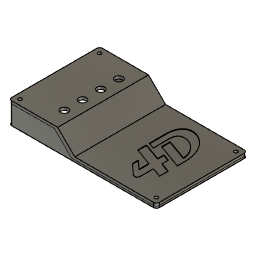
enclosure_top (Autodesk Fusion 360 design; units mm, degrees)
Autodesk Fusion 360 part; units mm, degrees
note: some values were not read from the file. Set by a fixed rule: which sketch regions a step uses.
sketch "Skizze1" plane through (0, 0, 0) normal (0, 0, 1) x (1, 0, 0)
  line L0 (0, 0) -> (130, 0)
  line L1 (130, 0) -> (130, 80)
  line L2 (130, 80) -> (0, 80)
  line L3 (0, 80) -> (0, 0)
  dimension "d1" = 80
  dimension "d2" = 130
  constraint horizontal L0
  constraint vertical L1
  constraint horizontal L2
  constraint vertical L3
  constraint coincident L0.start L3.end
  measures "d1" distance of L0.start L2.end
  measures "d2" distance of L0.start L0.end
extrude "Extrusion1" add sketch "Skizze1" along normal blind 19
sketch "Skizze2" plane through (0, 0, 0) normal (0, -1, 0) x (1, 0, 0)
  line L0 (0, 0) -> (130, 0)
  line L1 (130, 0) -> (130, 19)
  line L2 (130, 19) -> (0, 19)
  line L3 (0, 19) -> (0, 0)
  line L4 (0, 15) -> (40, 15)
  line L5 (40, 15) -> (55, 0)
  line L6 (55, 0) -> (0, 0)
  line L7 (0, 15) -> (0, 0)
  line L8 (43.0711, 19) -> (130, 19)
  line L9 (130, 19) -> (130, 4)
  line L10 (130, 4) -> (58.0711, 4)
  line L11 (58.0711, 4) -> (43.0711, 19)
  line L12 (47.5, 7.5) -> (51.0355, 11.0355) construction
  dimension "d5" = 15
  dimension "d6" = 40
  dimension "d7" = 45
  dimension "d8" = 135
  dimension "d10" = 4
  dimension "d11" = 5
  constraint coincident L3 L4.start
  constraint perpendicular L3 L4
  constraint coincident L0 L5.end
  constraint coincident L0.start L3.end
  constraint coincident L2 L8.start
  constraint coincident L1.end L2.start
  constraint perpendicular L1 L8
  constraint coincident L1 L9.end
  constraint perpendicular L8 L9
  constraint perpendicular L9 L10
  constraint midpoint L5 L12.start
  constraint perpendicular L5 L12
  constraint coincident L11 L12.end
  measures "d5" distance of L4.start L0.start
  measures "d6" distance of L4.start L4.end
  measures "d7" angle of L5 L6
  measures "d8" angle of L10 L11
  measures "d10" distance of L0.end L9.end
  measures "d11" distance of L12.start L12.end
extrude "Extrusion2" cut sketch "Skizze2" against normal blind 80 contours L0 L3 L4 L5 L6 L7 | L1 L2 L8 L9 L10 L11
shell "Schale1" thickness 2.5 removed faces 3 at (80, 53.3333, 0) at (45, 26.6667, 10) at (13.3333, 26.6667, 15)
sketch "Skizze3" plane through (0, 0, 0) normal (0, 0, -1) x (1, 0, 0)
  line L0 (127.5, -77.5) -> (55, -77.5)
  line L1 (55, -77.5) -> (55, -80)
  line L2 (55, -80) -> (130, -80)
  line L3 (130, -80) -> (130, 0)
  line L4 (130, 0) -> (55, 0)
  line L5 (55, 0) -> (55, -2.5)
  line L6 (55, -2.5) -> (127.5, -2.5)
  line L7 (127.5, -2.5) -> (127.5, -77.5)
  line L8 (55, 13.7) -> (135, 13.7)
  line L9 (135, 13.7) -> (135, -93.7)
  line L10 (135, -93.7) -> (55, -93.7)
  line L11 (55, -1.3) -> (127.5, -1.3)
  line L12 (128.7, -2.5) -> (128.7, -77.5)
  line L13 (127.5, -78.7) -> (55, -78.7)
  line L14 (55, 13.7) -> (55, -1.3)
  line L15 (55, -78.7) -> (55, -93.7)
  arc A0 (128.7, -2.5) -> (127.5, -1.3) centre (127.5, -2.5) ccw
  arc A1 (127.5, -78.7) -> (128.7, -77.5) centre (127.5, -77.5) ccw
  dimension "d16" = 1.3
  dimension "d17" = 1.3
  dimension "d20" = 1.3
  dimension "d21" = 15
  dimension "d22" = 80
  constraint horizontal L8
  constraint vertical L9
  constraint horizontal L10
  constraint horizontal L11
  constraint vertical L12
  constraint horizontal L13
  constraint vertical L14
  constraint vertical L15
  constraint vertical L11.start L13.end
  constraint equal L14 L15
  constraint coincident L5 L11.start
  constraint tangent L11 A0
  constraint tangent L12 A0
  constraint tangent L12 A1
  constraint tangent L13 A1
  constraint equal A0 A1
  constraint coincident L6.end L7.start
  measures "d16" distance of L4 L11.start
  measures "d17" distance of L1.end L13.end
  measures "d20" distance of L3 L12.start
  measures "d21" distance of L8.start L11.start
  measures "d22" distance of L8.start L8.end
extrude "Extrusion3" cut sketch "Skizze3" against normal blind 1.5 contours L1 L2 L3 L4 L5 L11 L12 L13 L14 L15 A0 A1
sketch "Skizze4" plane through (0, 0, 15) normal (0, 0, -1) x (1, 0, 0)
  line L0 (2.5, -77.5) -> (2.5, -2.5)
  line L1 (0, 0) -> (0, -80)
  line L2 (40, 8.7) -> (-10, 8.7)
  line L3 (-10, 8.7) -> (-10, -88.7)
  line L4 (-10, -88.7) -> (40, -88.7)
  line L5 (2.5, -1.3) -> (40, -1.3)
  line L6 (40, -78.7) -> (2.5, -78.7)
  line L7 (1.3, -77.5) -> (1.3, -2.5)
  line L8 (40, 8.7) -> (40, -1.3)
  line L9 (40, -88.7) -> (40, -78.7)
  line L10 (40, 0) -> (55, 0)
  line L11 (55, -80) -> (40, -80)
  arc A0 (2.5, -1.3) -> (1.3, -2.5) centre (2.5, -2.5) ccw
  arc A1 (1.3, -77.5) -> (2.5, -78.7) centre (2.5, -77.5) ccw
  point P0 (40, -2.5)
  dimension "d75" = 1.3
  dimension "d76" = 1.3
  dimension "d77" = 1.3
  dimension "d79" = 50
  dimension "d80" = 10
  constraint horizontal L2
  constraint vertical L3
  constraint horizontal L4
  constraint horizontal L5
  constraint horizontal L6
  constraint vertical L7
  constraint vertical L8
  constraint vertical L9
  constraint vertical L5.end L6.start
  constraint coincident L8 P0
  constraint tangent L5 A0
  constraint tangent L7 A0
  constraint tangent L6 A1
  constraint tangent L7 A1
  constraint equal A0 A1
  constraint coincident L0.end A0.centre
  constraint equal L8 L9
  measures "d75" distance of L5.end L10
  measures "d76" distance of L6.start L11
  measures "d77" distance of L1.start L7
  measures "d79" distance of L2.start L2.end
  measures "d80" distance of L2.start L5.end
extrude "Extrusion4" cut sketch "Skizze4" against normal blind 1.5
sketch "Skizze6" plane through (0, 80, 0) normal (0, 1, 0) x (-1, 0, 0)
  line L0 (-130, 1.5) -> (-55, 1.5)
  line L1 (-55, 1.5) -> (-55, 0)
  line L2 (-55, 0) -> (-40, 15)
  line L3 (-40, 16.5) -> (-55, 1.5)
  line L4 (-55, 1.5) -> (-55, 0)
  line L5 (-55, 0) -> (-40, 15)
  line L6 (-40, 15) -> (-40, 16.5)
  line L7 (-40, 16.5) -> (0, 16.5)
  line L8 (0, 16.5) -> (0, 19)
  line L9 (0, 19) -> (-43.0711, 19)
  line L10 (-43.0711, 19) -> (-58.0711, 4)
  line L11 (-58.0711, 4) -> (-130, 4)
  line L12 (-130, 4) -> (-130, 1.5)
  line L13 (-40, 15) -> (-40, 16.5)
  constraint coincident L3.start L6.end
  constraint coincident L0.end L1.start
  constraint perpendicular L0 L4
  constraint coincident L2.end L5.end
  constraint parallel L2 L5
extrude "Extrusion6" cut sketch "Skizze6" against normal blind 1.3 contours L1 L2 L3 L4 L5 L6 L13
sketch "Skizze7" plane through (0, 0, 0) normal (0, -1, 0) x (1, 0, 0)
  line L0 (40, 15) -> (55, 0)
  line L1 (55, 0) -> (55, 1.5)
  line L2 (55, 1.5) -> (130, 1.5)
  line L3 (40, 16.5) -> (55, 1.5)
  line L4 (55, 1.5) -> (55, 0)
  line L5 (55, 0) -> (40, 15)
  line L6 (40, 15) -> (40, 16.5)
  line L7 (0, 16.5) -> (40, 16.5)
  line L8 (130, 1.5) -> (130, 4)
  line L9 (130, 4) -> (58.0711, 4)
  line L10 (58.0711, 4) -> (43.0711, 19)
  line L11 (43.0711, 19) -> (0, 19)
  line L12 (0, 19) -> (0, 16.5)
  line L13 (40, 16.5) -> (40, 15)
  constraint coincident L3.start L6.end
  constraint coincident L1.end L2.start
  constraint coincident L0.end L1.start
  constraint coincident L0.start L5.end
extrude "Extrusion7" cut sketch "Skizze7" against normal blind 1.3 contours L0 L1 L3 L4 L5 L6 L13
sketch "Skizze8" plane through (0, 0, 19) normal (0, 0, 1) x (-1, 0, 0)
  circle A0 centre (-33, -64) radius 3.35
  circle A1 centre (-33, -48) radius 3.35
  circle A2 centre (-33, -32) radius 3.35
  circle A3 centre (-33, -16) radius 3.35
  line L0 (-43.0711, 0) -> (-43.0711, -80)
  line L1 (-43.0711, -80) -> (0, -80)
  line L2 (0, -80) -> (0, 0)
  dimension "d40" = 16
  dimension "d41" = 16
  dimension "d42" = 16
  dimension "d69" = 33
  dimension "d70" = 64
  dimension "d71" = 6.7
  constraint vertical A0.centre A1.centre
  constraint vertical A1.centre A2.centre
  constraint vertical A2.centre A3.centre
  constraint equal A0 A1
  constraint equal A1 A2
  constraint equal A2 A3
  measures "d40" distance of A0.centre A1.centre
  measures "d41" distance of A1.centre A2.centre
  measures "d42" distance of A2.centre A3.centre
  measures "d69" distance of A3.centre L2
  measures "d70" distance of A3.centre L1
  measures "d71" diameter of A3
extrude "Extrusion8" cut sketch "Skizze8" against normal blind 2.5
sketch "Skizze14" plane through (0, 0, 4) normal (0, 0, 1) x (-1, 0, 0)
  circle A0 centre (-125, -75) radius 1.55
  circle A1 centre (-125, -5) radius 1.55
  line L0 (-58.0711, 0) -> (-130, 0)
  line L1 (-130, 0) -> (-130, -80)
  line L2 (-130, -80) -> (-58.0711, -80)
  line L3 (-58.0711, -80) -> (-58.0711, 0)
  dimension "d62" = 3.1
  dimension "d72" = 5
  dimension "d73" = 5
  dimension "d74" = 5
  constraint equal A0 A1
  constraint vertical A0.centre A1.centre
  measures "d62" diameter of A1
  measures "d72" distance of A1.centre L0
  measures "d73" distance of A1.centre L1
  measures "d74" distance of A0.centre L2
extrude "Extrusion11" cut sketch "Skizze14" against normal blind 3 contours A0 | A1
sketch "Skizze16" plane through (0, 0, 19) normal (0, 0, 1) x (-1, 0, 0)
  line L0 (0, 0) -> (-43.0711, 0)
  line L1 (-43.0711, 0) -> (-43.0711, -80)
  line L2 (-43.0711, -80) -> (0, -80)
  line L3 (0, -80) -> (0, 0)
  circle A0 centre (-33, -32) radius 3.35
  circle A1 centre (-33, -48) radius 3.35
  circle A2 centre (-33, -16) radius 3.35
  circle A3 centre (-33, -64) radius 3.35
  circle A4 centre (-5, -75) radius 1.55
  circle A5 centre (-5, -5) radius 1.55
  dimension "d82" = 5
  dimension "d83" = 5
  dimension "d84" = 5
  dimension "d85" = 3.1
  constraint equal A4 A5
  constraint vertical A4.centre A5.centre
  measures "d82" distance of L2 A4.centre
  measures "d83" distance of L0 A5.centre
  measures "d84" distance of L3 A4.centre
  measures "d85" diameter of A4
extrude "Extrusion13" cut sketch "Skizze16" against normal blind 3 contours A4 | A5
fillet "Abrundung3" radius 2.5 4 edges at (0, 80, 17.75) (0, 0, 17.75) (130, 80, 2.75) (130, 0, 2.75)
sketch "Skizze17" plane through (90, 40, 4) normal (0, 0, 1) x (1, 0, 0)
  line L0 (-1.4651, -14.4481) -> (5.796, -21.0157)
  line L1 (5.796, -21.0157) -> (5.796, -12.5255)
  line L2 (5.796, -12.5255) -> (-9.4519, -6.9418)
  line L3 (-9.4519, -6.9418) -> (-9.4519, 0.6678)
  line L4 (-9.4519, 0.6678) -> (5.796, -4.6582)
  line L5 (5.796, -4.6582) -> (5.796, 0.8324)
  line L6 (5.796, 0.8324) -> (11.7734, -1.3438)
  line L7 (11.7734, -1.3438) -> (11.7734, -6.7557)
  line L8 (11.7734, -6.7557) -> (20.056, -9.7766)
  line L9 (20.056, -9.7766) -> (20.056, -17.329)
  line L10 (20.056, -17.329) -> (11.7734, -14.3725)
  line L11 (11.7734, -14.3725) -> (11.7734, -25.318)
  spline S0 degree 3 poles (11.7734, -25.318) (11.7734, -25.318) (11.7734, -25.3181) (11.7734, -25.3183) (11.7734, -25.3186) (11.7734, -25.319) (11.7734, -25.3196) (11.7734, -25.3202) (11.7734, -25.3211) (11.7734, -25.3225) (11.7734, -25.3242) (11.7734, -25.3263) (11.7734, -25.3284) (11.7734, -25.3311) (11.7734, -25.3346) (11.7734, -25.3387) (11.7734, -25.3442) (11.7733, -25.3511) (11.7733, -25.3594) (11.7733, -25.3676) (11.7732, -25.3759) (11.7731, -25.3868) (11.773, -25.4005) (11.7728, -25.4169) (11.7726, -25.4332) (11.7723, -25.4549) (11.7718, -25.4819) (11.7711, -25.5141) (11.7702, -25.5462) (11.7692, -25.5782) (11.7681, -25.6099) (11.7664, -25.6519) (11.764, -25.7039) (11.7606, -25.7659) (11.7567, -25.8271) (11.7522, -25.8876) (11.7456, -25.967) (11.736, -26.0645) (11.7223, -26.1794) (11.7066, -26.2915) (11.6887, -26.4008) (11.6688, -26.5073) (11.6467, -26.6111) (11.6149, -26.7444) (11.5699, -26.9043) (11.507, -27.0872) (11.4357, -27.2591) (11.3559, -27.4199) (11.2677, -27.5697) (11.1711, -27.7084) (11.066, -27.8361) (10.9524, -27.9526) (10.8305, -28.058) (10.7001, -28.1523) (10.5614, -28.2354) (10.4144, -28.3073) (10.259, -28.3681) (10.0953, -28.4178) (9.9234, -28.4563) (9.7747, -28.479) (9.6518, -28.4917) (9.5567, -28.4986) (9.4761, -28.502) (9.4107, -28.5034) (9.3624, -28.5037) (9.3155, -28.5034) (9.2551, -28.5018) (9.18, -28.4981) (9.0904, -28.4905) (8.972, -28.4765) (8.8254, -28.4513) (8.6518, -28.4091) (8.4807, -28.3549) (8.3121, -28.2888) (8.1459, -28.2107) (7.9247, -28.0896) (7.6528, -27.9069) (7.4496, -27.7365) (7.3494, -27.6446) knots 0 0 0 0 0.00001294 0.00002592 0.00005187 0.00010377 0.00015567 0.00020756 0.00031133 0.00041508 0.00062254 0.00082993 0.00103725 0.00124451 0.00165881 0.00207285 0.00248661 0.00331332 0.00413896 0.00496351 0.00578698 0.00660938 0.00825093 0.00988818 0.01152113 0.01314978 0.01639424 0.01962161 0.02283196 0.02602533 0.02920179 0.03236141 0.03863031 0.04483256 0.05096866 0.05703916 0.0630446 0.07486244 0.08642708 0.09774361 0.10881742 0.11965428 0.13026033 0.14064212 0.16075931 0.18006878 0.19863963 0.21654934 0.23388415 0.25073894 0.26721674 0.28342762 0.29948697 0.31551328 0.33162563 0.34794105 0.36457213 0.38162506 0.39919822 0.41738144 0.42672863 0.43625795 0.44597816 0.45091257 0.45589776 0.46045281 0.46499147 0.47402494 0.48300989 0.49195782 0.50978616 0.52760499 0.54550558 0.56357677 0.5819037 0.60056686 0.63918115 0.6799679 0.6799679 0.6799679 0.6799679
  line L12 (7.3494, -27.6446) -> (-1.4651, -19.5553)
  line L13 (-1.4651, -19.5553) -> (-1.4651, -14.4481)
  spline S1 degree 3 poles (0.3411, 31.4964) (2.9039, 31.4964) (5.6027, 30.6087) (8.459, 28.8334) knots 0 0 0 0 0.055556 0.055556 0.055556 0.055556
  spline S2 degree 3 poles (8.459, 28.8334) (8.4591, 28.8333) (8.4595, 28.8331) (8.4601, 28.8327) (8.4611, 28.8321) (8.4627, 28.8311) (8.4645, 28.83) (8.467, 28.8284) (8.47, 28.8265) (8.4737, 28.8242) (8.4773, 28.8219) (8.4822, 28.8189) (8.4883, 28.815) (8.4957, 28.8104) (8.5054, 28.8043) (8.5177, 28.7966) (8.5323, 28.7874) (8.5469, 28.7782) (8.5616, 28.7689) (8.581, 28.7566) (8.6054, 28.7412) (8.6346, 28.7226) (8.6637, 28.7039) (8.7025, 28.6791) (8.7509, 28.6478) (8.8089, 28.6102) (8.8667, 28.5724) (8.9244, 28.5344) (8.982, 28.4963) (9.0585, 28.4452) (9.1538, 28.3809) (9.2677, 28.303) (9.381, 28.2245) (9.4938, 28.1452) (9.6434, 28.0387) (9.8291, 27.9037) (10.0497, 27.739) (10.2681, 27.5715) (10.4844, 27.4013) (10.6984, 27.2283) (10.9102, 27.0526) (11.1898, 26.8145) (11.5339, 26.5099) (11.9379, 26.1334) (12.3331, 25.7458) (12.7196, 25.3472) (13.0972, 24.9375) (13.5903, 24.375) (14.1851, 23.6434) (14.8619, 22.7233) (15.5035, 21.7589) (16.1101, 20.7501) (16.6815, 19.697) (17.0356, 18.9728) (17.2068, 18.6037) knots 0 0 0 0 0.000054 0.000108 0.000216 0.000433 0.000649 0.000865 0.001298 0.001731 0.002164 0.002596 0.003462 0.004327 0.005192 0.006923 0.008653 0.010383 0.012113 0.013843 0.017303 0.020761 0.02422 0.027677 0.034591 0.041502 0.048411 0.055318 0.062224 0.069127 0.082928 0.096723 0.110512 0.124294 0.138072 0.165615 0.193145 0.220666 0.248184 0.275701 0.303224 0.330757 0.385869 0.441074 0.49641 0.551911 0.607615 0.663556 0.77628 0.890366 1.006077 1.123665 1.243373 1.365427 1.365427 1.365427 1.365427
  spline S3 degree 3 poles (17.2068, 18.6037) (17.2069, 18.6035) (17.207, 18.6032) (17.2073, 18.6025) (17.2079, 18.6013) (17.2087, 18.5997) (17.2096, 18.5977) (17.2108, 18.595) (17.2124, 18.5916) (17.2148, 18.5862) (17.2179, 18.5795) (17.2216, 18.5714) (17.2253, 18.5634) (17.2302, 18.5526) (17.2364, 18.5391) (17.2437, 18.523) (17.2535, 18.5015) (17.2658, 18.4745) (17.2804, 18.4422) (17.295, 18.4099) (17.3096, 18.3775) (17.329, 18.3344) (17.3531, 18.2804) (17.3819, 18.2156) (17.4105, 18.1507) (17.4485, 18.0642) (17.4956, 17.9559) (17.5515, 17.8258) (17.6068, 17.6954) (17.6615, 17.5649) (17.7155, 17.4341) (17.7868, 17.2596) (17.8743, 17.0409) (17.9768, 16.7776) (18.077, 16.5135) (18.1746, 16.2487) (18.3015, 15.8946) (18.454, 15.4499) (18.6271, 14.9131) (18.7903, 14.3731) (18.9437, 13.83) (19.0872, 13.2837) (19.2208, 12.7342) (19.386, 11.9967) (19.5677, 11.0663) (19.746, 9.9383) (19.8846, 8.7975) (19.9836, 7.644) (20.043, 6.4778) (20.056, 5.6958) (20.056, 5.303) knots 0 0 0 0 0.000055 0.000111 0.000222 0.000444 0.000666 0.000888 0.001332 0.001775 0.002663 0.003551 0.004438 0.005326 0.007101 0.008876 0.010651 0.0142 0.017749 0.021297 0.024845 0.028393 0.035486 0.042578 0.049668 0.056757 0.070928 0.085093 0.099252 0.113406 0.127553 0.141696 0.169966 0.198219 0.226457 0.254682 0.282897 0.339305 0.3957 0.452103 0.508531 0.565005 0.621544 0.678166 0.791733 0.905863 1.020705 1.136407 1.253112 1.370963 1.370963 1.370963 1.370963
  line L14 (20.056, 5.303) -> (20.056, -1.6194)
  line L15 (20.056, -1.6194) -> (-1.4629, 5.9759)
  line L16 (-1.4629, 5.9759) -> (-1.4629, 13.5497)
  line L17 (-1.4629, 13.5497) -> (16.6986, 7.107)
  spline S4 degree 3 poles (16.6986, 7.107) (16.6986, 7.1071) (16.6986, 7.1073) (16.6986, 7.1078) (16.6986, 7.1086) (16.6986, 7.1097) (16.6986, 7.111) (16.6986, 7.1128) (16.6986, 7.1151) (16.6986, 7.1187) (16.6986, 7.1231) (16.6986, 7.1285) (16.6986, 7.1339) (16.6986, 7.1411) (16.6985, 7.1501) (16.6985, 7.1608) (16.6984, 7.1752) (16.6983, 7.1931) (16.6982, 7.2146) (16.698, 7.2362) (16.6978, 7.2577) (16.6974, 7.2864) (16.6969, 7.3223) (16.6961, 7.3653) (16.6953, 7.4083) (16.6939, 7.4657) (16.6918, 7.5374) (16.6888, 7.6234) (16.6852, 7.7094) (16.6811, 7.7954) (16.6764, 7.8814) (16.6694, 7.996) (16.6594, 8.1393) (16.6451, 8.3111) (16.6286, 8.4828) (16.6099, 8.6544) (16.582, 8.8833) (16.5416, 9.1694) (16.4844, 9.5121) (16.4183, 9.8546) (16.3435, 10.1968) (16.2598, 10.5387) (16.1674, 10.8803) (16.0319, 11.337) (15.8402, 11.9077) (15.5757, 12.5891) (15.276, 13.2694) (14.941, 13.9487) (14.5709, 14.6269) (14.3036, 15.0735) (14.1644, 15.2965) knots 0 0 0 0 0.000034 0.000067 0.000135 0.000269 0.000404 0.000538 0.000807 0.001077 0.001615 0.002153 0.002691 0.00323 0.004306 0.005383 0.006459 0.008612 0.010765 0.012917 0.01507 0.017222 0.021527 0.025832 0.030136 0.03444 0.043048 0.051656 0.060264 0.068873 0.077483 0.086094 0.103322 0.120559 0.137809 0.155074 0.172357 0.206989 0.241726 0.276593 0.311609 0.346798 0.382181 0.417778 0.489693 0.562709 0.636979 0.712648 0.789854 0.868727 0.868727 0.868727 0.868727
  spline S5 degree 3 poles (14.1644, 15.2965) (14.1642, 15.2967) (14.164, 15.2972) (14.1634, 15.298) (14.1627, 15.2991) (14.1619, 15.3005) (14.1608, 15.3022) (14.1594, 15.3044) (14.1572, 15.3079) (14.1545, 15.3123) (14.1511, 15.3176) (14.1478, 15.3229) (14.1434, 15.3299) (14.1379, 15.3387) (14.1312, 15.3493) (14.1224, 15.3633) (14.1113, 15.3808) (14.0979, 15.4018) (14.0846, 15.4228) (14.0712, 15.4437) (14.0534, 15.4716) (14.0311, 15.5064) (14.0042, 15.548) (13.9773, 15.5895) (13.9413, 15.6447) (13.8962, 15.7133) (13.8418, 15.7953) (13.7871, 15.8767) (13.7322, 15.9577) (13.677, 16.0383) (13.6031, 16.1449) (13.5102, 16.2769) (13.3975, 16.4337) (13.2837, 16.5886) (13.169, 16.7415) (13.015, 16.9425) (12.8199, 17.189) (12.5811, 17.4779) (12.3382, 17.7592) (12.0913, 18.0329) (11.8402, 18.2989) (11.585, 18.5574) (11.2404, 18.8909) (10.799, 19.2892) (10.2513, 19.7381) (9.6871, 20.1566) (9.1064, 20.5446) (8.5093, 20.9021) (8.1004, 21.12) (7.8935, 21.2238) knots 0 0 0 0 0.000078 0.000156 0.000312 0.000468 0.000624 0.000936 0.001247 0.001871 0.002494 0.003118 0.003741 0.004987 0.006233 0.007478 0.009967 0.012455 0.014941 0.017425 0.019908 0.024869 0.029823 0.03477 0.039712 0.049574 0.059412 0.069224 0.079011 0.088773 0.098511 0.117913 0.13722 0.156433 0.175555 0.194587 0.232391 0.269861 0.307014 0.343869 0.380443 0.416755 0.452823 0.524301 0.59504 0.665201 0.734951 0.804461 0.873901 0.873901 0.873901 0.873901
  spline S6 degree 3 poles (7.8935, 21.2238) (7.8934, 21.2238) (7.8932, 21.2239) (7.8929, 21.2241) (7.8922, 21.2244) (7.8914, 21.2249) (7.8903, 21.2254) (7.8889, 21.2262) (7.8871, 21.2271) (7.8842, 21.2285) (7.8806, 21.2303) (7.8763, 21.2325) (7.872, 21.2347) (7.8663, 21.2376) (7.8592, 21.2412) (7.8506, 21.2455) (7.8392, 21.2513) (7.8249, 21.2585) (7.8078, 21.2671) (7.7908, 21.2757) (7.7737, 21.2843) (7.7509, 21.2957) (7.7226, 21.3099) (7.6886, 21.3268) (7.6546, 21.3437) (7.6095, 21.366) (7.5532, 21.3937) (7.4858, 21.4266) (7.4187, 21.4592) (7.3518, 21.4913) (7.2851, 21.5231) (7.1968, 21.565) (7.087, 21.6163) (6.9558, 21.6767) (6.8255, 21.7356) (6.6963, 21.793) (6.526, 21.8673) (6.3156, 21.9565) (6.0656, 22.0583) (5.8194, 22.1544) (5.577, 22.2446) (5.3384, 22.329) (5.1036, 22.4075) (4.799, 22.5035) (4.4276, 22.6093) (3.992, 22.7145) (3.6376, 22.7836) (3.362, 22.8268) (3.1614, 22.8531) (2.9645, 22.8735) (2.8028, 22.8857) (2.6754, 22.8926) (2.5813, 22.8962) (2.5034, 22.898) (2.4417, 22.8988) (2.3859, 22.899) (2.3208, 22.8987) (2.2217, 22.8979) (2.099, 22.8957) (1.9531, 22.8914) (1.7619, 22.8833) (1.5273, 22.8689) (1.2512, 22.8446) (0.9821, 22.8133) (0.6366, 22.7628) (0.2216, 22.6828) (-0.254, 22.5575) (-0.7013, 22.4042) (-1.1203, 22.2226) (-1.5109, 22.0128) (-1.873, 21.7746) (-2.2063, 21.5081) (-2.5108, 21.2133) (-2.6938, 20.9987) (-2.7801, 20.8873) knots 0 0 0 0 0.00003005 0.00006014 0.00012032 0.00024068 0.00036103 0.00048137 0.00072202 0.00096264 0.00144376 0.00192474 0.00240557 0.00288625 0.00384717 0.0048075 0.00576724 0.00768497 0.00960035 0.01151337 0.01342405 0.01533238 0.01914201 0.02294226 0.02673314 0.03051466 0.03804964 0.04554728 0.05300764 0.06043079 0.06781679 0.07516572 0.0897526 0.10419204 0.11848461 0.13263093 0.14663163 0.1741986 0.20119112 0.22761498 0.25347635 0.27878182 0.30353842 0.32775366 0.37459045 0.41936519 0.46215919 0.48284361 0.5030689 0.52284881 0.54219807 0.55171634 0.56113294 0.57044998 0.5750719 0.57966975 0.58716436 0.59461529 0.609387 0.62398697 0.63841733 0.66677752 0.69448674 0.72156503 0.74803394 0.79923121 0.84828989 0.89544477 0.94096141 0.98513626 1.02829475 1.0707871 1.11298145 1.15525519 1.15525519 1.15525519 1.15525519
  spline S7 degree 3 poles (-2.7801, 20.8873) (-2.7802, 20.8872) (-2.7803, 20.887) (-2.7806, 20.8866) (-2.7812, 20.8859) (-2.7819, 20.885) (-2.7828, 20.8838) (-2.784, 20.8822) (-2.7855, 20.8803) (-2.7873, 20.8779) (-2.7892, 20.8756) (-2.7916, 20.8724) (-2.7946, 20.8685) (-2.7982, 20.8638) (-2.803, 20.8575) (-2.809, 20.8496) (-2.8161, 20.8401) (-2.8233, 20.8306) (-2.8304, 20.8211) (-2.8399, 20.8083) (-2.8517, 20.7923) (-2.8658, 20.773) (-2.8798, 20.7536) (-2.8984, 20.7275) (-2.9215, 20.6947) (-2.9488, 20.6549) (-2.9759, 20.6147) (-3.0026, 20.5741) (-3.0291, 20.533) (-3.064, 20.4776) (-3.1069, 20.4072) (-3.157, 20.3212) (-3.206, 20.2336) (-3.2537, 20.1442) (-3.316, 20.0222) (-3.3909, 19.8654) (-3.4754, 19.6714) (-3.5551, 19.4706) (-3.6299, 19.2631) (-3.6999, 19.0488) (-3.765, 18.8278) (-3.8463, 18.5207) (-3.9353, 18.1195) (-4.0216, 17.6165) (-4.0883, 17.0869) (-4.1357, 16.5305) (-4.1636, 15.9474) (-4.1692, 15.5498) (-4.1689, 15.3466) knots 0 0 0 0 0.000037 0.000074 0.000148 0.000296 0.000444 0.000592 0.000889 0.001185 0.001481 0.001778 0.002371 0.002964 0.003558 0.004745 0.005934 0.007124 0.008315 0.009506 0.011893 0.014284 0.016678 0.019077 0.023888 0.028716 0.033563 0.038428 0.043312 0.048215 0.058083 0.068033 0.078071 0.0882 0.098422 0.119161 0.140314 0.161905 0.183955 0.206486 0.229517 0.253065 0.301779 0.352753 0.406095 0.461894 0.520233 0.581178 0.581178 0.581178 0.581178
  line L18 (-4.1689, 15.3466) -> (-4.1501, 1.3928)
  line L19 (-4.1501, 1.3928) -> (-9.4345, 3.1323)
  line L20 (-9.4345, 3.1323) -> (-9.4519, 18.6037)
  spline S8 degree 3 poles (-9.4519, 18.6037) (-9.4519, 18.6038) (-9.4519, 18.6041) (-9.4519, 18.6047) (-9.4519, 18.6057) (-9.4519, 18.6071) (-9.4519, 18.6088) (-9.4519, 18.6111) (-9.4519, 18.614) (-9.4519, 18.6185) (-9.4519, 18.6242) (-9.4519, 18.6311) (-9.4519, 18.6379) (-9.4519, 18.6471) (-9.4519, 18.6585) (-9.4519, 18.6721) (-9.4518, 18.6904) (-9.4518, 18.7131) (-9.4517, 18.7404) (-9.4515, 18.7677) (-9.4514, 18.7949) (-9.4511, 18.8312) (-9.4507, 18.8765) (-9.4501, 18.9308) (-9.4494, 18.985) (-9.4483, 19.057) (-9.4465, 19.1469) (-9.444, 19.2544) (-9.441, 19.3615) (-9.4375, 19.4683) (-9.4335, 19.5747) (-9.4275, 19.7157) (-9.4189, 19.8912) (-9.4065, 20.1005) (-9.3922, 20.3083) (-9.376, 20.5145) (-9.3519, 20.7866) (-9.3169, 21.123) (-9.2671, 21.5218) (-9.2095, 21.9146) (-9.1442, 22.3012) (-9.0711, 22.6817) (-8.9903, 23.0561) (-8.8728, 23.5446) (-8.7068, 24.1406) (-8.4754, 24.8351) (-8.2129, 25.5051) (-7.9194, 26.1507) (-7.5948, 26.7717) (-7.3568, 27.1708) (-7.2328, 27.3659) knots 0 0 0 0 0.000043 0.000086 0.000171 0.000342 0.000514 0.000685 0.001027 0.00137 0.002055 0.002739 0.003424 0.004108 0.005476 0.006843 0.00821 0.010942 0.013672 0.016399 0.019124 0.021847 0.027285 0.032714 0.038133 0.043543 0.054335 0.065089 0.075807 0.086488 0.097133 0.107741 0.12885 0.149818 0.170645 0.191333 0.211886 0.252592 0.292778 0.332462 0.371664 0.410401 0.448694 0.486563 0.561108 0.634218 0.706081 0.776895 0.846865 0.916207 0.916207 0.916207 0.916207
  spline S9 degree 3 poles (-7.2328, 27.3659) (-7.2327, 27.366) (-7.2326, 27.3662) (-7.2323, 27.3667) (-7.2319, 27.3672) (-7.2315, 27.3679) (-7.2309, 27.3688) (-7.2302, 27.3699) (-7.2291, 27.3717) (-7.2277, 27.374) (-7.226, 27.3767) (-7.2242, 27.3793) (-7.222, 27.3829) (-7.2191, 27.3874) (-7.2157, 27.3928) (-7.2111, 27.3999) (-7.2054, 27.4089) (-7.1985, 27.4196) (-7.1916, 27.4303) (-7.1847, 27.4409) (-7.1755, 27.4551) (-7.164, 27.4729) (-7.1501, 27.4941) (-7.1362, 27.5153) (-7.1176, 27.5434) (-7.0944, 27.5784) (-7.0663, 27.6203) (-7.0381, 27.6619) (-7.0098, 27.7033) (-6.9813, 27.7444) (-6.9433, 27.799) (-6.8954, 27.8666) (-6.8374, 27.9469) (-6.7788, 28.0263) (-6.7198, 28.1048) (-6.6406, 28.208) (-6.5403, 28.3349) (-6.4178, 28.4838) (-6.2932, 28.6292) (-6.1666, 28.7709) (-6.038, 28.909) (-5.9074, 29.0436) (-5.7311, 29.2177) (-5.5055, 29.4266) (-5.2261, 29.6635) (-4.9385, 29.8861) (-4.6429, 30.0942) (-4.3392, 30.288) (-4.0275, 30.4674) (-3.7076, 30.6324) (-3.2693, 30.8337) (-2.6991, 31.0498) (-1.9846, 31.2504) (-1.2379, 31.3932) (-0.4591, 31.4784) (0.0713, 31.4964) (0.3411, 31.4964) knots 0 0 0 0 0.00004 0.00008 0.000159 0.000239 0.000319 0.000478 0.000638 0.000957 0.001276 0.001594 0.001913 0.002551 0.003188 0.003825 0.005098 0.006371 0.007643 0.008914 0.010184 0.012723 0.015258 0.01779 0.02032 0.02537 0.030408 0.035435 0.04045 0.045453 0.050446 0.060396 0.070303 0.080167 0.089988 0.099768 0.119207 0.138492 0.157631 0.176631 0.1955 0.214247 0.23288 0.269836 0.30644 0.342764 0.378882 0.414868 0.450799 0.48675 0.522797 0.595462 0.669399 0.745166 0.82328 0.904213 0.904213 0.904213 0.904213
  line L21 (40, 37.5) -> (40, -37.5)
extrude "Extrusion14" cut sketch "Skizze17" against normal blind 0.5
sketch "Skizze18" plane through (0, 0, 16.5) normal (0, 0, -1) x (1, 0, 0)
  arc A0 (2.5, 0) -> (0, -2.5) centre (2.5, -2.5) ccw
  line L0 (0, -2.5) -> (0, -77.5)
  arc A1 (0, -77.5) -> (2.5, -80) centre (2.5, -77.5) ccw
  line L1 (2.5, -80) -> (40, -80)
  line L2 (40, -80) -> (40, -78.7)
  line L3 (40, -78.7) -> (2.5, -78.7)
  arc A2 (1.3, -77.5) -> (2.5, -78.7) centre (2.5, -77.5) ccw
  line L4 (1.3, -77.5) -> (1.3, -2.5)
  arc A3 (2.5, -1.3) -> (1.3, -2.5) centre (2.5, -2.5) ccw
  line L5 (2.5, -1.3) -> (40, -1.3)
  line L6 (40, -1.3) -> (40, 0)
  line L7 (40, 0) -> (2.5, 0)
  line L8 (2.5, -0.4) -> (40, -0.4)
  line L9 (40, -79.6) -> (2.5, -79.6)
  line L10 (0.4, -77.5) -> (0.4, -2.5)
  line L11 (2.5, 0) -> (40, 0)
  line L12 (40, -80) -> (2.5, -80)
  line L13 (0, -77.5) -> (0, -2.5)
  line L14 (40, 0) -> (40, -0.4)
  line L15 (40, -80) -> (40, -79.6)
  line L16 (0, -13) -> (0.4, -13) construction
  arc A4 (2.5, -0.4) -> (0.4, -2.5) centre (2.5, -2.5) ccw
  arc A5 (0.4, -77.5) -> (2.5, -79.6) centre (2.5, -77.5) ccw
  arc A6 (2.5, 0) -> (0, -2.5) centre (2.5, -2.5) ccw
  arc A7 (0, -77.5) -> (2.5, -80) centre (2.5, -77.5) ccw
  dimension "d95" = 0.4
  constraint horizontal L8
  constraint horizontal L9
  constraint vertical L10
  constraint horizontal L11
  constraint horizontal L12
  constraint vertical L13
  constraint vertical L14
  constraint vertical L15
  constraint vertical L8.end L9.start
  constraint equal L14 L15
  constraint coincident L13 L16.start
  constraint coincident L10 L16.end
  constraint perpendicular L10 L16
  constraint equal L14 L16
  constraint tangent L8 A4
  constraint tangent L10 A4
  constraint tangent L9 A5
  constraint tangent L10 A5
  constraint equal A4 A5
  constraint tangent L11 A6
  constraint tangent L13 A6
  constraint tangent L12 A7
  constraint tangent L13 A7
  constraint equal A6 A7
  constraint coincident L6.end L7.start
  constraint coincident L1.end L2.start
  constraint coincident L0 A0.end
  constraint coincident A0.centre A3.centre
  measures "d95" distance of L8.end L6.end
extrude "Extrusion15" add sketch "Skizze18" along normal blind 16.5 contours A0 L0 A1 L1 L2 L6 L7 L8 L9 L10 L11 L12 L13 L14 L15 A4 A5 A6 A7
sketch "Skizze19" plane through (0, 0, 15) normal (0, 0, -1) x (1, 0, 0)
  line L0 (40, -1.3) -> (2.5, -1.3)
  arc A0 (2.5, -1.3) -> (1.3, -2.5) centre (2.5, -2.5) ccw
  line L1 (1.3, -2.5) -> (1.3, -77.5)
  arc A1 (1.3, -77.5) -> (2.5, -78.7) centre (2.5, -77.5) ccw
  line L2 (2.5, -78.7) -> (40, -78.7)
  line L3 (40, -78.7) -> (40, -77.5)
  line L4 (40, -77.5) -> (2.5, -77.5)
  line L5 (2.5, -77.5) -> (2.5, -2.5)
  line L6 (2.5, -2.5) -> (40, -2.5)
  line L7 (40, -2.5) -> (40, -1.3)
  line L8 (40, -1.3) -> (2.5, -1.3)
  line L9 (1.3, -2.5) -> (1.3, -77.5)
  line L10 (2.5, -78.7) -> (40, -78.7)
  line L11 (40, -1.7) -> (2.5, -1.7)
  line L12 (1.7, -2.5) -> (1.7, -77.5)
  line L13 (2.5, -78.3) -> (40, -78.3)
  line L14 (40, -1.3) -> (40, -1.7)
  line L15 (40, -78.3) -> (40, -78.7)
  arc A2 (2.5, -1.3) -> (1.3, -2.5) centre (2.5, -2.5) ccw
  arc A3 (1.3, -77.5) -> (2.5, -78.7) centre (2.5, -77.5) ccw
  arc A4 (2.5, -1.7) -> (1.7, -2.5) centre (2.5, -2.5) ccw
  arc A5 (1.7, -77.5) -> (2.5, -78.3) centre (2.5, -77.5) ccw
  line L16 (1.3, -40) -> (1.7, -40) construction
  dimension "d100" = 0.4
  constraint horizontal L8
  constraint vertical L9
  constraint horizontal L10
  constraint horizontal L11
  constraint vertical L12
  constraint horizontal L13
  constraint perpendicular L8 L14
  constraint perpendicular L10 L15
  constraint vertical L11.start L13.end
  constraint tangent L8 A2
  constraint tangent L9 A2
  constraint tangent L9 A3
  constraint tangent L10 A3
  constraint equal A2 A3
  constraint tangent L11 A4
  constraint tangent L12 A4
  constraint tangent L12 A5
  constraint tangent L13 A5
  constraint equal A4 A5
  constraint midpoint L9 L16.start
  constraint coincident L12 L16.end
  constraint perpendicular L12 L16
  constraint equal L14 L16
  constraint equal L14 L15
  constraint coincident L0.start L7.end
  constraint coincident L2.end L3.start
  constraint coincident L1 A0.end
  constraint coincident A0.centre L5.end
  measures "d100" distance of L16.start L16.end
extrude "Extrusion16" add sketch "Skizze19" along normal blind 15 contours L0 A0 L1 A1 L2 L3 L7 L8 L9 L10 L11 L12 L13 L14 L15 A2 A3 A4 A5
sketch "Skizze20" plane through (0, 0, 1.5) normal (0, 0, -1) x (1, 0, 0)
  circle A0 centre (125, -75) radius 1.55
  circle A1 centre (125, -5) radius 1.55
  line L0 (127.5, -2.5) -> (57.0355, -2.5)
  line L1 (57.0355, -2.5) -> (57.0355, -77.5)
  line L2 (57.0355, -77.5) -> (127.5, -77.5)
  line L3 (127.5, -77.5) -> (127.5, -2.5)
  line L4 (57.0355, -2.5) -> (59.5355, -2.5)
  line L5 (59.5355, -2.5) -> (59.5355, -77.5)
  line L6 (59.5355, -77.5) -> (57.0355, -77.5)
  line L7 (57.0355, -77.5) -> (57.0355, -2.5)
  dimension "d103" = 2.5
  constraint horizontal L4
  constraint vertical L5
  constraint horizontal L6
  constraint vertical L7
  constraint coincident L0.end L1.start
  measures "d103" distance of L0.end L4.end
extrude "Extrusion17" add sketch "Skizze20" along normal blind 1.5 contours L0 L1 L2 L4 L5 L6 L7
sketch "Skizze21" plane through (0, 1.3, 0) normal (0, -1, 0) x (1, 0, 0)
  line L0 (55, 0) -> (127.5, 0)
  line L1 (127.5, 0) -> (127.5, 1.5)
  line L2 (127.5, 1.5) -> (55, 1.5)
  line L3 (55, 1.5) -> (40, 16.5)
  line L4 (40, 16.5) -> (2.5, 16.5)
  line L5 (2.5, 16.5) -> (2.5, 0)
  line L6 (2.5, 0) -> (40, 0)
  line L7 (40, 0) -> (40, 15)
  line L8 (40, 15) -> (55, 0)
  line L9 (40, 15) -> (40, 0)
  line L10 (40, 0) -> (55, 0)
  line L11 (55, 0) -> (40, 15)
  constraint coincident L7.end L8.start
  constraint coincident L6.end L7.start
  constraint coincident L0.start L8.end
extrude "Extrusion18" add sketch "Skizze21" against normal blind 0.4 contours L7 L8 L9 L10 L11
sketch "Skizze22" plane through (0, 0, 1.5) normal (0, 0, -1) x (1, 0, 0)
  arc A0 (130, -2.5) -> (127.5, 0) centre (127.5, -2.5) ccw
  line L0 (127.5, 0) -> (55, 0)
  line L1 (55, 0) -> (55, -1.3)
  line L2 (55, -1.3) -> (127.5, -1.3)
  arc A1 (128.7, -2.5) -> (127.5, -1.3) centre (127.5, -2.5) ccw
  line L3 (128.7, -2.5) -> (128.7, -77.5)
  arc A2 (127.5, -78.7) -> (128.7, -77.5) centre (127.5, -77.5) ccw
  line L4 (127.5, -78.7) -> (55, -78.7)
  line L5 (55, -78.7) -> (55, -80)
  line L6 (55, -80) -> (127.5, -80)
  arc A3 (127.5, -80) -> (130, -77.5) centre (127.5, -77.5) ccw
  line L7 (130, -77.5) -> (130, -2.5)
  line L8 (55, 0) -> (127.5, 0)
  line L9 (130, -2.5) -> (130, -77.5)
  line L10 (127.5, -80) -> (55, -80)
  arc A4 (130, -2.5) -> (127.5, 0) centre (127.5, -2.5) ccw
  arc A5 (127.5, -80) -> (130, -77.5) centre (127.5, -77.5) ccw
  line L11 (55, -0.4) -> (127.5, -0.4)
  line L12 (129.6, -2.5) -> (129.6, -77.5)
  line L13 (127.5, -79.6) -> (55, -79.6)
  arc A6 (129.6, -2.5) -> (127.5, -0.4) centre (127.5, -2.5) ccw
  arc A7 (127.5, -79.6) -> (129.6, -77.5) centre (127.5, -77.5) ccw
  line L14 (55, -0.4) -> (55, 0)
  line L15 (55, -80) -> (55, -79.6)
  dimension "d110" = 0.4
  dimension "d111" = 0.4
  constraint horizontal L8
  constraint vertical L9
  constraint horizontal L10
  constraint coincident L0.end L1.start
  constraint coincident L5.end L6.start
  constraint tangent L8 A4
  constraint tangent L9 A4
  constraint tangent L9 A5
  constraint tangent L10 A5
  constraint equal A4 A5
  constraint coincident A0.centre A1.centre
  constraint horizontal L11
  constraint vertical L12
  constraint horizontal L13
  constraint tangent L11 A6
  constraint tangent L12 A6
  constraint tangent L12 A7
  constraint tangent L13 A7
  constraint equal A6 A7
  constraint vertical L0.end L11.start
  constraint vertical L11.start L13.end
  constraint equal L14 L15
  measures "d110" distance of L0.end L11.start
  measures "d111" horizontal distance of A0.start L12.start
extrude "Extrusion19" add sketch "Skizze22" along normal blind 1.5 contours A0 L0 L1 L5 L6 A3 L7 L8 L9 L10 A4 A5 L11 L12 L13 A6 A7 L14 L15
sketch "Skizze23" plane through (0, 0, 0) normal (0, -1, 0) x (1, 0, 0)
  line L0 (127.5, 0) -> (127.5, 4)
  line L1 (127.5, 4) -> (58.0711, 4)
  line L2 (58.0711, 4) -> (43.0711, 19)
  line L3 (43.0711, 19) -> (2.5, 19)
  line L4 (2.5, 19) -> (2.5, 0)
  line L5 (2.5, 0) -> (40, 0)
  line L6 (40, 0) -> (40, 16.5)
  line L7 (40, 16.5) -> (55, 1.5)
  line L8 (55, 1.5) -> (55, 0)
  line L9 (55, 0) -> (127.5, 0)
  line L10 (40, 16.5) -> (40, 0)
  line L11 (40, 0) -> (55, 0)
  line L12 (55, 0) -> (55, 1.5)
  line L13 (55, 1.5) -> (40, 16.5)
  constraint coincident L6.end L7.start
  constraint coincident L5.end L6.start
  constraint coincident L8.end L9.start
  constraint coincident L7.end L8.start
extrude "Extrusion20" add sketch "Skizze23" against normal blind 0.4 contours L6 L7 L8 L10 L11 L12 L13
sketch "Skizze24" plane through (0, 78.7, 0) normal (0, 1, 0) x (-1, 0, 0)
  line L0 (-127.5, 0) -> (-55, 0)
  line L1 (-55, 0) -> (-40, 15)
  line L2 (-40, 15) -> (-40, 0)
  line L3 (-40, 0) -> (-2.5, 0)
  line L4 (-2.5, 0) -> (-2.5, 16.5)
  line L5 (-2.5, 16.5) -> (-40, 16.5)
  line L6 (-40, 16.5) -> (-55, 1.5)
  line L7 (-55, 1.5) -> (-127.5, 1.5)
  line L8 (-127.5, 1.5) -> (-127.5, 0)
  line L9 (-55, 0) -> (-40, 15)
  line L10 (-40, 15) -> (-40, 0)
  line L11 (-40, 0) -> (-55, 0)
  constraint coincident L0.end L1.start
  constraint coincident L1.end L2.start
  constraint coincident L2.end L3.start
extrude "Extrusion21" add sketch "Skizze24" against normal blind 0.4 contours L1 L2 L9 L10 L11
sketch "Skizze25" plane through (0, 80, 0) normal (0, 1, 0) x (-1, 0, 0)
  line L0 (-127.5, 4) -> (-127.5, 0)
  line L1 (-127.5, 0) -> (-55, 0)
  line L2 (-55, 0) -> (-55, 1.5)
  line L3 (-55, 1.5) -> (-40, 16.5)
  line L4 (-40, 16.5) -> (-40, 0)
  line L5 (-40, 0) -> (-2.5, 0)
  line L6 (-2.5, 0) -> (-2.5, 19)
  line L7 (-2.5, 19) -> (-43.0711, 19)
  line L8 (-43.0711, 19) -> (-58.0711, 4)
  line L9 (-58.0711, 4) -> (-127.5, 4)
  line L10 (-40, 16.5) -> (-40, 0)
  line L11 (-40, 0) -> (-55, 0)
  line L12 (-55, 0) -> (-55, 1.5)
  line L13 (-55, 1.5) -> (-40, 16.5)
  constraint coincident L3.end L4.start
  constraint coincident L4.end L5.start
  constraint coincident L1.end L2.start
  constraint coincident L2.end L3.start
extrude "Extrusion22" add sketch "Skizze25" against normal blind 0.4 contours L2 L3 L4 L10 L11 L12 L13
sketch "Skizze26" plane through (0, 0, 15) normal (0, 0, -1) x (1, 0, 0)
  line L0 (2.5, -78.3) -> (40, -78.3)
  line L1 (40, -78.3) -> (40, -77.5)
  line L2 (40, -77.5) -> (2.5, -77.5)
  line L3 (2.5, -77.5) -> (2.5, -2.5)
  line L4 (2.5, -2.5) -> (40, -2.5)
  line L5 (40, -2.5) -> (40, -1.7)
  line L6 (40, -1.7) -> (2.5, -1.7)
  arc A0 (2.5, -1.7) -> (1.7, -2.5) centre (2.5, -2.5) ccw
  line L7 (1.7, -2.5) -> (1.7, -77.5)
  arc A1 (1.7, -77.5) -> (2.5, -78.3) centre (2.5, -77.5) ccw
  line L8 (2.5, -2.5) -> (40, -2.5)
  line L9 (40, -77.5) -> (2.5, -77.5)
  line L10 (2.5, -77.5) -> (2.5, -2.5)
  line L11 (2.5, -2.1) -> (40, -2.1)
  line L12 (40, -77.9) -> (2.5, -77.9)
  line L13 (2.1, -77.5) -> (2.1, -2.5)
  line L14 (40, -77.9) -> (40, -77.5)
  arc A2 (2.5, -2.1) -> (2.1, -2.5) centre (2.5, -2.5) ccw
  arc A3 (2.1, -77.5) -> (2.5, -77.9) centre (2.5, -77.5) ccw
  line L15 (40, -2.1) -> (40, -2.5)
  dimension "d122" = 0.4
  dimension "d123" = 0.4
  constraint horizontal L8
  constraint horizontal L9
  constraint vertical L10
  constraint coincident L1.end L2.start
  constraint coincident L3.end L4.start
  constraint horizontal L11
  constraint horizontal L12
  constraint vertical L13
  constraint tangent L11 A2
  constraint tangent L13 A2
  constraint tangent L12 A3
  constraint tangent L13 A3
  constraint equal A2 A3
  constraint coincident L4.end L5.start
  constraint vertical L15
  measures "d122" distance of L3.end L13.end
  measures "d123" distance of L1.end L12.start
extrude "Extrusion23" add sketch "Skizze26" along normal blind 15 contours L1 L2 L3 L4 L5 L8 L9 L10 L11 L12 L13 L14 A2 A3 L15
sketch "Skizze27" plane through (0, 2.5, 0) normal (0, 1, 0) x (-1, 0, 0)
  line L0 (-57.0355, 1.5) -> (-57.0355, 0)
  line L1 (-57.0355, 0) -> (-55, 0)
  line L2 (-55, 0) -> (-40, 15)
  line L3 (-40, 15) -> (-40, 0)
  line L4 (-40, 0) -> (-2.5, 0)
  line L5 (-2.5, 0) -> (-2.5, 16.5)
  line L6 (-2.5, 16.5) -> (-42.0355, 16.5)
  line L7 (-42.0355, 16.5) -> (-57.0355, 1.5)
  line L8 (-40, 15) -> (-40, 0)
  line L9 (-40, 0) -> (-55, 0)
  line L10 (-55, 0) -> (-40, 15)
  constraint coincident L2.end L3.start
  constraint coincident L3.end L4.start
  constraint coincident L1.end L2.start
extrude "Extrusion24" add sketch "Skizze27" against normal blind 0.4 contours L2 L3 L8 L9 L10
sketch "Skizze28" plane through (0, 77.5, 0) normal (0, -1, 0) x (1, 0, 0)
  line L0 (57.0355, 0) -> (57.0355, 1.5)
  line L1 (57.0355, 1.5) -> (42.0355, 16.5)
  line L2 (42.0355, 16.5) -> (2.5, 16.5)
  line L3 (2.5, 16.5) -> (2.5, 0)
  line L4 (2.5, 0) -> (40, 0)
  line L5 (40, 0) -> (40, 15)
  line L6 (40, 15) -> (55, 0)
  line L7 (55, 0) -> (57.0355, 0)
  line L8 (40, 15) -> (40, 0)
  line L9 (40, 0) -> (55, 0)
  line L10 (55, 0) -> (40, 15)
  constraint coincident L5.end L6.start
  constraint coincident L4.end L5.start
  constraint coincident L6.end L7.start
extrude "Extrusion25" add sketch "Skizze28" against normal blind 0.4 contours L5 L6 L8 L9 L10
